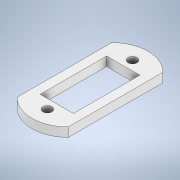
# Autodesk Inventor part: servo Holder
Saved by Autodesk Inventor 2021 (Build 250183000, 183)
## iProperties
Created: 2023-05-31
Part Number: servo Holder
Material: ABS Plastic
Document SubType Name: Modeling
Designer: shrus
Density: 1.06 g/cm^3
Appearance: Smooth - White
Author: shrus
Autodesk Inventor part; units mm, degrees
ref_plane "YZ Plane" through (0, 0, 0) normal (1, 0, 0) x (0, 1, 0)
ref_plane "XZ Plane" through (0, 0, 0) normal (0, 1, 0) x (-1, 0, 0)
ref_plane "XY Plane" through (0, 0, 0) normal (0, 0, 1) x (1, 0, 0)
sketch "Sketch1" plane through (0, 0, 0) normal (0, 1, 0) x (-1, 0, 0)
  line L0 (9.2564, 10.8677) -> (9.2564, -11.1323)
  line L1 (9.2564, -11.1323) -> (-1.7436, -11.1323)
  line L2 (-1.7436, -11.1323) -> (-1.7436, 10.8677)
  line L3 (-1.7436, 10.8677) -> (9.2564, 10.8677)
  line L4 (12.2564, -15.8323) -> (12.2564, 15.5677)
  line L5 (-4.7436, 15.5677) -> (-4.7436, -15.8323)
  arc A0 (12.2564, 15.5677) -> (-4.7436, 15.5677) centre (3.7564, 7.0972) ccw
  arc A1 (-4.7436, -15.8323) -> (12.2564, -15.8323) centre (3.7564, -7.3617) ccw
  circle A2 centre (3.7564, 13.9677) radius 1.5
  circle A3 centre (3.7564, -14.2323) radius 1.5
  point P0 (0, 0)
  dimension "d0" = 22
  constraints: 12 end point, 4 centre point, 4 point on circle, 3 perpendicular, 1 vertical
  measures "d0" distance of L0.start L0.end
extrude "Extrusion1" add sketch "Sketch1" along normal blind 3
body "Solid1"
